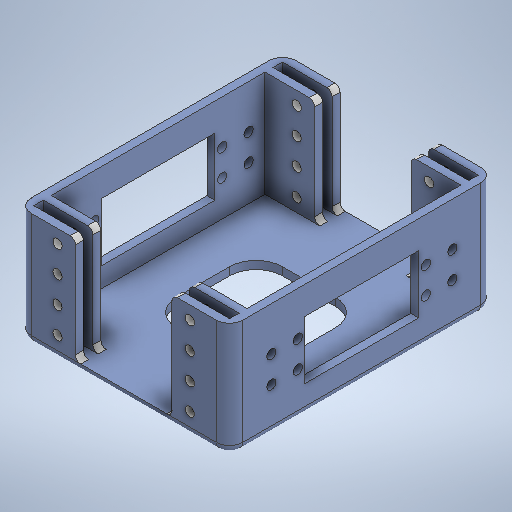
# Autodesk Inventor part: chassis
Saved by Autodesk Inventor 2025 (Build 290162000, 162)
## iProperties
Created: 2024-09-04
Part Number: chassis
Material: Générique
Document SubType Name: Modeling
Designer: chass
Density: 1 g/cm^3
Appearance: Par défaut
Author: chass
## iProperties of the stored document chassis_Impression 3D.ipt
Created: 2024-09-05
Part Number: chassis_Impression 3D
Material: Générique
Document SubType Name: Modeling
Designer: chass
Density: 1 g/cm^3
Appearance: Par défaut
Author: chass
Autodesk Inventor part; units mm, degrees
ref_plane "YZ Plane" through (0, 0, 0) normal (1, 0, 0) x (0, 1, 0)
ref_plane "XZ Plane" through (0, 0, 0) normal (0, 1, 0) x (-1, 0, 0)
ref_plane "XY Plane" through (0, 0, 0) normal (0, 0, 1) x (1, 0, 0)
sketch "Esquisse1" plane through (0, 0, 0) normal (0, 1, 0) x (-1, 0, 0)
  line L0 (40, 50) -> (-40, 50)
  line L1 (-40, 50) -> (-40, -50)
  line L2 (-40, -50) -> (40, -50)
  line L3 (40, -50) -> (40, 50)
  line L4 (40, 50) -> (-40, -50)
  line L5 (-40, 50) -> (40, -50)
  point P0 (0, 0)
  point P1 (0, 0)
  point P2 (0, 0)
  dimension "d73" = 80
  dimension "d74" = 100
  constraints: 12 end point, 2 midpoint, 2 parallel, 1 coincident, 1 horizontal, 1 perpendicular
  measures "d73" distance of L1.end L2.end
  measures "d74" distance of L0.end L1.end
extrude "Extrusion1" add sketch "Esquisse1" along normal blind 3
sketch "Esquisse2" plane through (0, 3, 0) normal (0, 1, 0) x (1, 0, 0)
  line L0 (-40, 50) -> (-40, -50) projected
  line L1 (40, 50) -> (-40, 50) projected
  line L2 (-40, -50) -> (-37, -50)
  line L3 (-37, -50) -> (-37, 50)
  line L4 (-37, 50) -> (-40, 50)
  line L5 (-40, 50) -> (-40, -50)
  line L6 (0, -93.4559) -> (0, 106.1011)
  line L7 (40, 50) -> (40, -50)
  line L8 (-40, 50) -> (40, 50)
  line L9 (40, -50) -> (37, -50)
  line L10 (37, -50) -> (37, 50)
  line L11 (-37, -50) -> (-18.25, -50)
  line L12 (-18.25, -50) -> (-18.25, -47)
  line L13 (-18.25, -47) -> (-37, -47)
  line L14 (-37, -47) -> (-37, -50)
  line L15 (-37, -43.4) -> (-18.25, -43.4)
  line L16 (-18.25, -43.4) -> (-18.25, -40.4)
  line L17 (-18.25, -40.4) -> (-37, -40.4)
  line L18 (-37, -40.4) -> (-37, -43.4)
  line L19 (-63.4161, 0) -> (50.7812, 0)
  line L20 (37, -50) -> (18.25, -50)
  line L21 (18.25, -50) -> (18.25, -47)
  line L22 (18.25, -47) -> (37, -47)
  line L23 (37, -47) -> (37, -50)
  line L24 (37, -43.4) -> (18.25, -43.4)
  line L25 (18.25, -43.4) -> (18.25, -40.4)
  line L26 (18.25, -40.4) -> (37, -40.4)
  line L27 (37, -40.4) -> (37, -43.4)
  line L28 (63.4161, 0) -> (-50.7812, 0)
  line L29 (-37, 50) -> (-18.25, 50)
  line L30 (-18.25, 50) -> (-18.25, 47)
  line L31 (-18.25, 47) -> (-37, 47)
  line L32 (-37, 47) -> (-37, 50)
  line L33 (-37, 43.4) -> (-18.25, 43.4)
  line L34 (-18.25, 43.4) -> (-18.25, 40.4)
  line L35 (-18.25, 40.4) -> (-37, 40.4)
  line L36 (-37, 40.4) -> (-37, 43.4)
  line L37 (18.25, 43.4) -> (18.25, 40.4)
  line L38 (18.25, 40.4) -> (37, 40.4)
  line L39 (18.25, 47) -> (37, 47)
  line L40 (18.25, 50) -> (18.25, 47)
  line L41 (37, 50) -> (18.25, 50)
  line L42 (37, 47) -> (37, 50)
  line L43 (37, 40.4) -> (37, 43.4)
  line L44 (37, 43.4) -> (18.25, 43.4)
  line L45 (40, -50) -> (40, 50) projected
  point P0 (0, 0)
  point P1 (37, 50)
  point P2 (-27.625, -47)
  point P3 (-27.625, -43.4)
  point P4 (27.625, -47)
  point P5 (27.625, -43.4)
  point P6 (-27.625, 47)
  point P7 (-27.625, 43.4)
  point P8 (27.625, 47)
  point P9 (27.625, 43.4)
  point P10 (37, 43.4)
  point P11 (37, 47)
  point P12 (18.25, 50)
  point P13 (-37, 43.4)
  point P14 (-37, 40.4)
  point P15 (-37, 47)
  point P16 (-18.25, 50)
  point P17 (37, -47)
  point P18 (37, -40.4)
  point P19 (-37, -47)
  dimension "d2" = 3
  dimension "d6" = 3
  dimension "d8" = 3
  dimension "d112" = 18.25
  dimension "d113" = 3.6
  constraints: 86 end point, 34 symmetric about line, 6 parallel, 4 horizontal, 3 perpendicular, 3 point on line, 2 midpoint, 1 collinear, 1 vertical
  measures "d2" distance of L4.end L3.end
  measures "d6" distance of L12.end L11.end
  measures "d8" distance of L15.end L16.end
  measures "d112" distance between parallel lines of L6 L12
  measures "d113" distance between parallel lines of L15 L13
extrude "Extrusion2" add sketch "Esquisse2" along normal blind 40 contours L1 L3 L19 L0 | L19 L3 L2 L0 | L1 L30 L31 L3 | L3 L13 L12 L11 | L17 L16 L15 L3 | L3 L33 L34 L35 | L19 L7 L9 L10 | L10 L1 L7 L19 | L1 L10 L39 L40 | L10 L24 L25 L26 | L38 L37 L44 L10 | L10 L20 L21 L22
sketch "Esquisse3" plane through (40, 0, 50) normal (1, 0, 0) x (0, 0, -1)
  line L0 (0, 0) -> (100, 0) projected
  line L1 (100, 0) -> (100, 43) projected
  line L2 (0, 3) -> (0, 43) projected
  line L3 (9.6, 43) -> (90.4, 43) projected
  line L4 (28.5, 32.5) -> (71.5, 32.5)
  line L5 (71.5, 32.5) -> (71.5, 10.5)
  line L6 (71.5, 10.5) -> (28.5, 10.5)
  line L7 (28.5, 10.5) -> (28.5, 32.5)
  line L8 (0, 43) -> (100, 0)
  line L9 (100, 43) -> (0, 0)
  line L10 (28.5, 10.5) -> (71.5, 32.5)
  line L11 (28.5, 32.5) -> (71.5, 10.5)
  line L12 (50, 43) -> (50, 0)
  circle A0 centre (25.8, 26.5) radius 1.75
  circle A1 centre (15.8, 26.5) radius 1.75
  line L13 (0, 21.5) -> (100, 21.5)
  circle A2 centre (15.8, 16.5) radius 1.75
  circle A3 centre (25.8, 16.5) radius 1.75
  circle A4 centre (84.2, 26.5) radius 1.75
  circle A5 centre (74.2, 26.5) radius 1.75
  circle A6 centre (84.2, 16.5) radius 1.75
  circle A7 centre (74.2, 16.5) radius 1.75
  point P0 (50, 21.5)
  point P1 (50, 21.5)
  point P2 (50, 21.5)
  dimension "d54" = 43
  dimension "d55" = 22
  dimension "d79" = 24.2
  dimension "d80" = 10
  dimension "d96" = 3.5
  dimension "d97" = 3.5
  dimension "d105" = 5
  constraints: 20 end point, 8 centre point, 6 midpoint, 6 symmetric about line, 3 parallel, 1 horizontal, 1 perpendicular, 1 point on line, 6 other
  measures "d54" distance of L5.end L6.end
  measures "d55" distance of L4.end L5.end
  measures "d79" distance from line of L12 A0.centre
  measures "d80" distance of A0.centre A1.centre
  measures "d96" diameter of A1
  measures "d97" diameter of A0
  measures "d105" distance from line of L13 A0.centre
extrude "Extrusion3" cut sketch "Esquisse3" against normal blind 100 contours L9 L10 L7 | L7 L13 L9 | L12 L11 L6 | L6 L10 L12 | L7 L8 L13 | L13 L5 L8 | L10 L5 L9 | L12 L4 L10 | L8 L7 L11 | L8 L5 L11 | L11 L4 L12 | L9 L5 L13 | A0 | A1 | A2 | A3 | A4 | A5 | A6 | A7
fillet "Congé1" radius 5 4 edges at (40, 21.5, 50) (-40, 21.5, 50) (40, 21.5, -50) (-40, 21.5, -50)
fillet "Congé2" radius 3 8 edges at (-38.5355, 0, 48.5355) (0, 0, 50) (38.5355, 0, 48.5355) (40, 0, 0) (38.5355, 0, -48.5355) (0, 0, -50) (-38.5355, 0, -48.5355) (-40, 0, 0)
sketch "Esquisse5" plane through (0, 3, 0) normal (0, 1, 0) x (1, 0, 0)
  line L0 (-20, -20) -> (20, -20)
  line L1 (20, -20) -> (20, 20)
  line L2 (20, 20) -> (-20, 20)
  line L3 (-20, 20) -> (-20, -20)
  line L4 (-20, -20) -> (20, 20)
  line L5 (20, -20) -> (-20, 20)
  point P0 (0, 0)
  point P1 (0, 0)
  point P2 (0, 0)
  dimension "d106" = 40
  dimension "d107" = 40
  constraints: 12 end point, 2 midpoint, 2 parallel, 1 coincident, 1 horizontal, 1 perpendicular
  measures "d106" distance of L2.end L0.start
  measures "d107" distance of L1.end L2.end
extrude "Extrusion5" cut sketch "Esquisse5" against normal blind 3
fillet "Congé5" radius 10 4 edges at (-20, 1.5, 20) (-20, 1.5, -20) (20, 1.5, 20) (20, 1.5, -20)
sketch "Esquisse6" plane through (-35, 43, 50) normal (0, 0, 1) x (1, 0, 0)
  circle A0 centre (10, -14.9609) radius 1.75
  line L0 (-5, 0) -> (-5, -40) projected
  line L1 (-5, 0) -> (75, 0)
  line L2 (75, 0) -> (75, -43)
  line L3 (75, -43) -> (-5, -43)
  line L4 (-5, -43) -> (-5, 0)
  line L5 (-5, -19.9609) -> (75, -19.9609)
  line L6 (35, -43) -> (35, 0)
  circle A1 centre (10, -4.9609) radius 1.75
  circle A2 centre (10, -24.9609) radius 1.75
  circle A3 centre (10, -34.9609) radius 1.75
  circle A4 centre (60, -14.9609) radius 1.75
  circle A5 centre (60, -4.9609) radius 1.75
  circle A6 centre (60, -24.9609) radius 1.75
  circle A7 centre (60, -34.9609) radius 1.75
  dimension "d114" = 3.5
  dimension "d115" = 5
  dimension "d116" = 25
  dimension "d117" = 3.5
  dimension "d118" = 10
  constraints: 12 end point, 8 centre point, 6 symmetric about line, 2 parallel, 2 perpendicular, 2 point on line, 1 horizontal, 1 midpoint, 6 other
  measures "d114" diameter of A0
  measures "d115" distance from line of L5 A0.centre
  measures "d116" distance from line of A0.centre L6
  measures "d117" diameter of A1
  measures "d118" distance of A0.centre A1.centre
extrude "Extrusion6" cut sketch "Esquisse6" against normal blind 115.75 contours A0 | A1 | A2 | A3 | A4 | A5 | A6 | A7
fillet "Congé6" radius 2 8 edges at (-18.25, 3, 41.9) (-18.25, 3, 48.5) (18.25, 3, 48.5) (18.25, 3, 41.9) (18.25, 3, -41.9) (18.25, 3, -48.5) (-18.25, 3, -48.5) (-18.25, 3, -41.9)
fillet "Congé7" radius 2 8 edges at (-18.25, 43, -48.5) (-18.25, 43, -41.9) (18.25, 43, -48.5) (18.25, 43, -41.9) (-18.25, 43, 41.9) (-18.25, 43, 48.5) (18.25, 43, 41.9) (18.25, 43, 48.5)
